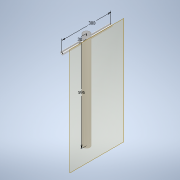
# Autodesk Inventor part: FrontWheelHandle
Saved by Autodesk Inventor 2022.2 (Build 262287000, 287)
## iProperties
Created: 2022-04-15
Part Number: FrontWheelHandle
Material: Aluminum 6061
Document SubType Name: Modeling
Designer: foriw
Density: 2.7 g/cm^3
Appearance: Aluminum - Flat
Author: foriw
Autodesk Inventor part; units mm, degrees
ref_plane "XZ Plane" through (0, 0, 0) normal (0, 1, 0) x (-1, 0, 0)
ref_plane "XY Plane" through (0, 0, 0) normal (0, 0, 1) x (1, 0, 0)
sketch "Sketch1" plane through (0, 0, 0) normal (1, 0, 0) x (0, 1, 0)
  line L0 (0, 0) -> (595, 0)
  line L1 (565, -150) -> (565, 150)
  point P0 (565, 0)
  dimension "d0" = 595
  dimension "d1" = 30
  dimension "d2" = 300
  constraints: 4 end point, 1 horizontal, 1 midpoint, 1 point on line, 1 vertical
  measures "d0" distance of L0.start L0.end
  measures "d1" distance of L0.end point (565, 0)
  measures "d2" distance of L1.start L1.end
sketch "Sketch2" plane through (0, 0, 0) normal (0, 1, 0) x (-1, 0, 0)
  circle A0 centre (0, 0) radius 21
  circle A1 centre (0, 0) radius 18
  dimension "d3" = 42
  dimension "d4" = 3
  constraints: 2 centre point, 1 coincident
  measures "d3" diameter of A0
  measures "d4" radial gap between concentric circles of A0 A1
ref_plane "Work Plane1" through (0, 565, 0) normal (0, 0, 1) x (1, 0, 0)
sketch "Sketch3" plane through (0, 565, 0) normal (0, 0, 1) x (1, 0, 0)
  circle A0 centre (0, 0) radius 10
  circle A1 centre (0, 0) radius 8
  point P0 (0, -565)
  dimension "d5" = 20
  dimension "d6" = 2
  constraints: 2 centre point
  measures "d5" diameter of A0
  measures "d6" radial gap between concentric circles of A0 A1
extrude "Extrusion1" add sketch "Sketch3" along normal mid plane 300
extrude "Extrusion2" add sketch "Sketch2" along normal up to surface (595 mm away)
ref_plane "Work Plane2" through (64, 0, 0) normal (1, 0, 0) x (0, 1, 0)
sketch "Sketch4" plane through (64, 0, 0) normal (1, 0, 0) x (0, 1, 0)
  circle A0 centre (16, 0) radius 2
  circle A1 centre (45, 0) radius 2
  line L0 (43, 7.4424) -> (43, -6.8322)
  line L1 (18, 4.2123) -> (18, -2.7864)
  line L2 (14, 2.9252) -> (14, -3.9898)
  line L3 (0, -21) -> (0, 21) projected
  point P0 (0, 0)
  dimension "d12" = 4
  dimension "d13" = 4
  dimension "d14" = 25
  dimension "d15" = 14
  constraints: 6 end point, 3 tangent, 3 vertical, 2 centre point
  measures "d12" diameter of A0
  measures "d13" diameter of A1
  measures "d14" distance between parallel lines of L0 L1
  measures "d15" distance between parallel lines of L3 L2
extrude "Extrusion3" cut sketch "Sketch4" against normal blind 54.75
equation "\"d13\" = d12"
body "Solid1"
